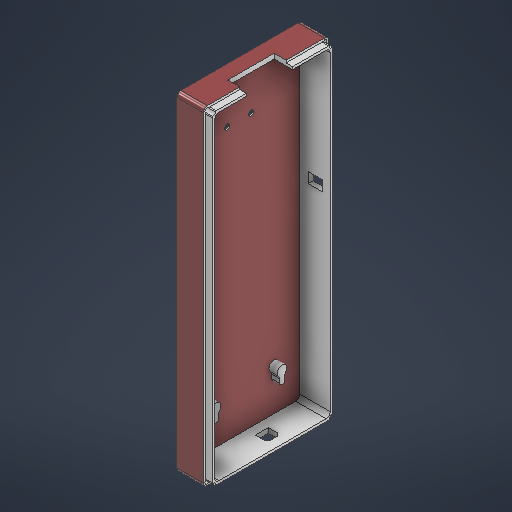
# Autodesk Inventor part: cDAQ_Bottom_Box3
Saved by Autodesk Inventor 2027 (Build 310192000, 192)
## iProperties
Created: 2026-05-08
Part Number: cDAQ_Bottom_Box3
Material: Generic
Document SubType Name: Modeling
Designer: giese
Density: 1 g/cm^3
Appearance: Default
Author: giese
Autodesk Inventor part; units mm, degrees
ref_plane "YZ Plane" through (0, 0, 0) normal (1, 0, 0) x (0, 1, 0)
ref_plane "XZ Plane" through (0, 0, 0) normal (0, 1, 0) x (-1, 0, 0)
ref_plane "XY Plane" through (0, 0, 0) normal (0, 0, 1) x (1, 0, 0)
sketch "Sketch1" plane through (0, 0, 0) normal (1, 0, 0) x (0, 1, 0)
  line L0 (37.5698, 48.0867) -> (-215.7952, 48.0867)
  line L1 (-215.7952, 48.0867) -> (-215.7952, -48.4333)
  line L2 (-215.7952, -48.4333) -> (37.5698, -48.4333)
  line L3 (37.5698, -48.4333) -> (37.5698, 48.0867)
  point P0 (0, 0)
  dimension "d0" = 96.52
  dimension "d1" = 253.365
  constraints: 8 end point, 2 parallel, 1 horizontal, 1 perpendicular
  measures "d0" distance of L2.end L0.start
  measures "d1" distance of L1.end L2.end
extrude "Extrusion1" add sketch "Sketch1" along normal blind 20.32
sketch "Sketch2" plane through (20.32, 0, 0) normal (1, 0, 0) x (0, 0, -1)
  line L0 (44.6233, 33.7598) -> (-44.2767, 33.7598)
  line L1 (-44.2767, 33.7598) -> (-44.2767, -211.9852)
  line L2 (-44.2767, -211.9852) -> (44.6233, -211.9852)
  line L3 (44.6233, -211.9852) -> (44.6233, 33.7598)
  line L4 (48.4333, 37.5698) -> (-48.0867, 37.5698) projected
  line L5 (-48.0867, 37.5698) -> (-48.0867, -215.7952) projected
  point P0 (0, 0)
  dimension "d4" = 245.745
  dimension "d5" = 88.9
  dimension "d8" = 3.81
  dimension "d21" = 3.81
  constraints: 8 end point, 2 parallel, 1 horizontal, 1 perpendicular
  measures "d4" distance of L2.end L0.start
  measures "d5" distance of L0.start L0.end
  measures "d8" distance between parallel lines of L0 L4
  measures "d21" distance between parallel lines of L5 L1
extrude "Extrusion2" cut sketch "Sketch2" against normal blind 18.415
sketch "Sketch3" plane through (0, 0, 0) normal (-1, 0, 0) x (0, 0, 1)
  circle A0 centre (-7.1989, -2.6638) radius 2
  circle A1 centre (11.2999, -2.6638) radius 2
  circle A2 centre (29.7987, -2.6638) radius 2
  line L0 (-48.4333, -215.7952) -> (-48.4333, 37.5698) projected
  line L1 (-48.4333, 37.5698) -> (48.0867, 37.5698) projected
  line L2 (48.0867, 37.5698) -> (48.0867, -215.7952) projected
  line L3 (44.2767, 33.7598) -> (-44.6233, 33.7598) projected
  point P0 (0, 0)
  point P1 (-0.896, -23.7433)
  point P2 (-45.1848, 27.0137)
  dimension "d9" = 18.4988
  dimension "d10" = 4
  dimension "d11" = 4
  dimension "d12" = 18.4988
  dimension "d13" = 36.9976
  dimension "d18" = 18.288
  dimension "d22" = 4
  dimension "d58" = 40.2336
  constraints: 3 centre point
  measures "d9" distance of A0.centre A1.centre
  measures "d10" diameter of A1
  measures "d11" diameter of A2
  measures "d12" distance of A1.centre A2.centre
  measures "d13" distance of A0.centre A2.centre
  measures "d18" distance from line of L2 A2.centre
  measures "d22" diameter of A0
  measures "d58" distance from line of L1 A2.centre
extrude "Extrusion3" cut sketch "Sketch3" against normal blind 3.81
sketch "Sketch5" plane through (0, -215.7952, -48.4333) normal (0, 0, -1) x (-1, 0, 0)
  line L0 (-19.2532, 150.6728) -> (-8.5598, 150.6728)
  line L1 (-8.5598, 150.6728) -> (-8.5598, 158.6728)
  line L2 (-8.5598, 158.6728) -> (-19.2532, 158.6728)
  line L3 (-19.2532, 158.6728) -> (-19.2532, 150.6728)
  line L4 (0, 253.365) -> (-20.32, 253.365) projected
  line L5 (0, 0) -> (0, 253.365) projected
  point P0 (0, 215.7952)
  point P1 (-13.9065, 158.6728)
  point P2 (-13.9065, 150.6728)
  dimension "d28" = 10.6934
  dimension "d30" = 8
  dimension "d31" = 8.5598
  dimension "d34" = 102.6922
  constraints: 8 end point, 2 midpoint, 2 parallel, 1 horizontal, 1 perpendicular
  measures "d28" distance between parallel lines of L1 L3
  measures "d30" distance of point (-13.907, 158.673) point (-13.907, 150.673)
  measures "d31" distance between parallel lines of L5 L1
  measures "d34" distance between parallel lines of L4 L0
extrude "Extrusion4" cut sketch "Sketch5" against normal blind 24.13
sketch "Sketch6" plane through (0, -215.7952, -48.4333) normal (0, -1, 0) x (1, 0, 0)
  line L0 (16, 45.1284) -> (9, 45.1284)
  line L1 (9, 45.1284) -> (9, 35.1284)
  line L2 (9, 35.1284) -> (16, 35.1284)
  line L3 (0, 96.52) -> (0, 0) projected
  line L4 (18.24, 43.1283) -> (18.24, 37.1284)
  line L5 (16, 45.1284) -> (18.24, 43.1283)
  line L6 (18.24, 37.1284) -> (16, 35.1284)
  line L7 (0, 0) -> (20.32, 0) projected
  point P0 (0, 48.4333)
  point P1 (12.5, 45.1284)
  point P2 (12.5, 35.1284)
  dimension "d35" = 10
  dimension "d39" = 6
  dimension "d48" = 45.1284
  dimension "d49" = 18.24
  constraints: 12 end point, 2 midpoint, 1 horizontal, 1 parallel, 1 perpendicular, 1 vertical
  measures "d35" distance of point (12.5, 45.128) point (12.5, 35.128)
  measures "d39" distance of L4.start L4.end
  measures "d48" distance between parallel lines of L7 L0
  measures "d49" distance between parallel lines of L3 L4
extrude "Extrusion5" cut sketch "Sketch6" against normal blind 3.81
sketch "Sketch7" plane through (0, 37.5698, 48.0867) normal (0, 1, 0) x (1, 0, 0)
  line L0 (26.1366, 63.754) -> (11.1252, 63.754)
  line L1 (11.1252, 63.754) -> (11.1252, 28.194)
  line L2 (11.1252, 28.194) -> (26.1366, 28.194)
  line L3 (26.1366, 28.194) -> (26.1366, 63.754)
  line L4 (0, 0) -> (20.32, 0) projected
  line L5 (0, 96.52) -> (0, 0) projected
  line L6 (20.32, 96.52) -> (20.32, 0) projected
  point P0 (0, 48.0867)
  dimension "d51" = 35.56
  dimension "d52" = 28.194
  dimension "d55" = 11.1252
  dimension "d56" = 15.0114
  dimension "d57" = 5.8166
  constraints: 8 end point, 2 parallel, 1 horizontal, 1 perpendicular
  measures "d51" distance of L2.end L0.start
  measures "d52" distance between parallel lines of L4 L2
  measures "d55" distance between parallel lines of L5 L1
  measures "d56" distance between parallel lines of L3 L1
  measures "d57" distance between parallel lines of L6 L3
extrude "Extrusion6" cut sketch "Sketch7" against normal blind 7.62
fillet "Fillet1" radius 3.175 4 edges at (10.16, 37.5698, -48.4333) (10.16, 37.5698, 48.0867) (10.16, -215.7952, -48.4333) (10.16, -215.7952, 48.0867)
sketch "Sketch8" plane through (0, 0, 0) normal (-1, 0, 0) x (0, 0, 1)
  line L0 (-8.9705, -6.1944) -> (-5.4399, -6.1944)
  line L1 (-8.9705, 0.8668) -> (-5.4399, 0.8668)
  line L2 (-8.9705, -6.1944) -> (-11.0089, -2.6638)
  line L3 (-8.9705, 0.8668) -> (-11.0089, -2.6638)
  line L4 (-5.4399, -6.1944) -> (-3.4016, -2.6638)
  line L5 (-5.4399, 0.8668) -> (-3.4016, -2.6638)
  circle A0 centre (-7.1989, -2.6638) radius 2 projected
  line L6 (9.5283, -6.1944) -> (13.0589, -6.1944)
  line L7 (9.5283, 0.8668) -> (13.0589, 0.8668)
  line L8 (9.5283, -6.1944) -> (7.4899, -2.6638)
  line L9 (9.5283, 0.8668) -> (7.4899, -2.6638)
  line L10 (13.0589, -6.1944) -> (15.0973, -2.6638)
  line L11 (13.0589, 0.8668) -> (15.0973, -2.6638)
  circle A1 centre (11.2999, -2.6638) radius 2 projected
  line L12 (28.0271, -6.1944) -> (25.9887, -2.6638)
  line L13 (28.0271, 0.8668) -> (25.9887, -2.6638)
  line L14 (28.0271, -6.1944) -> (31.5577, -6.1944)
  line L15 (28.0271, 0.8668) -> (31.5577, 0.8668)
  line L16 (31.5577, -6.1944) -> (33.5961, -2.6638)
  line L17 (31.5577, 0.8668) -> (33.5961, -2.6638)
  circle A2 centre (29.7987, -2.6638) radius 2 projected
  point P0 (-7.2052, -6.1944)
  point P1 (11.2936, -6.1944)
  point P2 (29.7924, -6.1944)
  point P3 (-11.0089, -2.6638)
  point P4 (-3.4016, -2.6638)
  point P5 (15.0973, -2.6638)
  point P6 (7.4899, -2.6638)
  point P7 (33.5961, -2.6638)
  point P8 (25.9887, -2.6638)
  dimension "d60" = 7.0612
  dimension "d61" = 120
  dimension "d62" = 120
  dimension "d63" = 120
  dimension "d64" = 120
  dimension "d65" = 3.5306
  dimension "d66" = 3.5306
  dimension "d67" = 3.5306
  dimension "d68" = 3.5306
  dimension "d69" = 3.5306
  dimension "d70" = 3.5306
  dimension "d71" = 0
  dimension "d72" = 7.6074
  dimension "d73" = 3.81
  dimension "d74" = 0
  dimension "d75" = 7.0612
  dimension "d76" = 120
  dimension "d77" = 120
  dimension "d78" = 120
  dimension "d79" = 120
  dimension "d80" = 3.5306
  dimension "d81" = 3.5306
  dimension "d82" = 3.5306
  dimension "d83" = 3.5306
  dimension "d84" = 3.5306
  dimension "d85" = 3.5306
  dimension "d86" = 0
  dimension "d87" = 7.6074
  dimension "d91" = 0
  dimension "d92" = 3.81
  dimension "d93" = 7.0612
  dimension "d94" = 120
  dimension "d95" = 120
  dimension "d96" = 120
  dimension "d97" = 120
  dimension "d98" = 3.5306
  dimension "d99" = 3.5306
  dimension "d100" = 3.5306
  dimension "d101" = 3.5306
  dimension "d102" = 3.5306
  dimension "d103" = 3.5306
  dimension "d104" = 0
  dimension "d105" = 7.6074
  dimension "d108" = 0
  dimension "d109" = 3.81
  constraints: 36 end point, 6 horizontal, 3 midpoint
  measures "d60" distance from line of point (-7.205, -6.194) L1
  measures "d61" angle of L0 L2
  measures "d62" angle of L1 L3
  measures "d63" angle of L4 L0
  measures "d64" angle of L5 L1
  measures "d65" distance of L0.start L0.end
  measures "d66" distance of L1.start L1.end
  measures "d67" vertical distance of L1.start L3.end
  measures "d68" vertical distance of L0.start L2.end
  measures "d69" vertical distance of L1.end L5.end
  measures "d70" vertical distance of L0.end L4.end
  measures "d71" horizontal distance of L0.start L1.start
  measures "d72" distance of L4.end L2.end
  measures "d73" distance of A0.centre L2.end
  measures "d74" vertical distance of A0.centre L4.end
  measures "d75" distance from line of point (11.294, -6.194) L7
  measures "d76" angle of L6 L8
  measures "d77" angle of L7 L9
  measures "d78" angle of L10 L6
  measures "d79" angle of L11 L7
  measures "d80" distance of L8.start L6.end
  measures "d81" distance of L9.start L7.end
  measures "d82" vertical distance of L9.start L9.end
  measures "d83" vertical distance of L8.start L8.end
  measures "d84" vertical distance of L7.end L11.end
  measures "d85" vertical distance of L6.end L10.end
  measures "d86" horizontal distance of L8.start L9.start
  measures "d87" distance of L10.end L8.end
  measures "d91" vertical distance of A1.centre L8.end
  measures "d92" distance of A1.centre L8.end
  measures "d93" distance from line of point (29.792, -6.194) L15
  measures "d94" angle of L14 L12
  measures "d95" angle of L15 L13
  measures "d96" angle of L16 L14
  measures "d97" angle of L17 L15
  measures "d98" distance of L12.start L16.start
  measures "d99" distance of L15.start L15.end
  measures "d100" vertical distance of L15.start L13.end
  measures "d101" vertical distance of L12.start L12.end
  measures "d102" vertical distance of L15.end L17.end
  measures "d103" vertical distance of L16.start L16.end
  measures "d104" horizontal distance of L12.start L15.start
  measures "d105" distance of L16.end L12.end
  measures "d108" vertical distance of A2.centre L12.end
  measures "d109" distance of A2.centre L12.end
extrude "Extrusion7" cut sketch "Sketch8" against normal blind 0.9525 contours L2 L3 L1 L5 L4 L0 | A0 | L8 L9 L7 L11 L10 L6 | A1 | L12 L13 L15 L17 L16 L14 | A2
sketch "Sketch9" plane through (1.905, 0, 0) normal (1, 0, 0) x (0, 0, -1)
  arc A0 (27.3489, -182.3284) -> (21.8927, -182.3284) centre (24.6208, -179.8542) ccw
  line L0 (45.2583, 37.5698) -> (15.6673, 37.5698) projected
  line L1 (44.6233, 33.7598) -> (44.6233, -211.9852) projected
  arc A1 (22.7158, -187.4742) -> (26.5258, -187.4742) centre (24.6208, -187.4742) ccw
  line L2 (26.5258, -187.4742) -> (26.5258, -184.4614)
  line L3 (22.7158, -187.4742) -> (22.7158, -184.4614)
  arc A2 (27.3489, -182.3284) -> (26.5258, -184.4614) centre (29.7008, -184.4614) ccw
  arc A3 (22.7158, -184.4614) -> (21.8927, -182.3284) centre (19.5408, -184.4614) ccw
  arc A4 (-23.4511, -182.3284) -> (-28.9073, -182.3285) centre (-26.1792, -179.8542) ccw
  arc A5 (-28.0842, -187.4606) -> (-24.2742, -187.4742) centre (-26.1792, -187.4742) ccw
  line L4 (-24.2742, -187.4742) -> (-24.2742, -184.4614)
  line L5 (-28.0842, -187.4606) -> (-28.0842, -184.4614)
  arc A6 (-23.4511, -182.3284) -> (-24.2742, -184.4614) centre (-21.0992, -184.4614) ccw
  arc A7 (-28.0842, -184.4614) -> (-28.9073, -182.3285) centre (-31.2592, -184.4614) ccw
  line L6 (-19.8927, 37.5698) -> (-44.9117, 37.5698) projected
  line L7 (-44.2767, -211.9852) -> (-44.2767, 33.7598) projected
  point P0 (0, 0)
  point P1 (26.5258, -183.0063)
  point P2 (22.7158, -183.0063)
  point P3 (-24.2742, -183.0063)
  point P4 (-28.0842, -183.0063)
  dimension "d112" = 217.424
  dimension "d114" = 7.366
  dimension "d116" = 3.81
  dimension "d117" = 225.044
  dimension "d118" = 3.175
  dimension "d119" = 7.366
  dimension "d120" = 3.81
  dimension "d121" = 3.175
  dimension "d122" = 217.424
  dimension "d123" = 225.044
  dimension "d125" = 0
  dimension "d128" = 50.8
  dimension "d129" = 20.0025
  dimension "d130" = 0
  constraints: 20 point on circle, 8 centre point, 8 end point, 8 tangent, 4 point on line, 2 equal radius, 2 parallel, 2 vertical
  measures "d112" distance from line of L0 A0.centre
  measures "d114" diameter of A0
  measures "d116" diameter of A1
  measures "d117" distance from line of L0 A1.centre
  measures "d118" radius of A2
  measures "d119" diameter of A4
  measures "d120" diameter of A5
  measures "d121" radius of A6
  measures "d122" distance from line of A4.centre L6
  measures "d123" distance from line of L6 A5.centre
  measures "d125" horizontal distance of A5.centre A4.centre
  measures "d128" distance of A5.centre A1.centre
  measures "d129" distance from line of L1 A0.centre
  measures "d130" horizontal distance of A0.centre A1.centre
extrude "Extrusion8" add sketch "Sketch9" along normal blind 6.4008
sketch "Sketch10" plane through (20.32, 0, 0) normal (1, 0, 0) x (0, 0, -1)
  line L0 (44.6233, -211.9852) -> (-44.2767, -211.9852) projected
  line L1 (-44.2767, -211.9852) -> (-44.2767, 33.7598) projected
  line L2 (-44.2767, -211.9852) -> (-44.2767, -209.6992)
  line L3 (-46.2767, -211.4452) -> (-46.2767, -213.9852)
  line L4 (-46.2767, -213.9852) -> (-41.9907, -213.9852)
  line L5 (-44.2767, -211.9852) -> (-41.9907, -211.9852)
  line L6 (44.6233, -211.9852) -> (42.3373, -211.9852)
  line L7 (42.3373, -213.9852) -> (46.6233, -213.9852)
  line L8 (46.6233, -213.9852) -> (46.6233, -209.6992)
  line L9 (44.6233, 33.7598) -> (44.6233, -211.9852) projected
  line L10 (-44.2767, -209.6992) -> (-44.2767, 33.7598)
  line L11 (-44.2767, 33.7598) -> (44.6233, 33.7598) projected
  line L12 (-41.9907, 35.7598) -> (-46.2767, 35.7598)
  line L13 (-46.2767, 35.7598) -> (-46.2767, 29.7278)
  line L14 (42.3373, 33.7598) -> (44.6233, 33.7598)
  line L15 (46.6233, 31.4738) -> (46.6233, 35.7598)
  line L16 (46.6233, 35.7598) -> (42.3373, 35.7598)
  line L17 (-41.9907, -213.9852) -> (42.3373, -213.9852)
  line L18 (42.3373, -211.9852) -> (-41.9907, -211.9852)
  line L19 (46.6233, -209.6992) -> (46.6233, 31.4738)
  line L20 (44.6233, 31.4738) -> (44.6233, -209.6992)
  line L21 (42.3373, 33.7598) -> (-41.9907, 33.7598)
  line L22 (-41.9907, 35.7598) -> (42.3373, 35.7598)
  line L23 (-44.2767, -209.6992) -> (-44.2767, -209.6992)
  line L24 (-46.2767, 29.7278) -> (-46.2767, -211.4452)
  point P0 (-41.9907, -213.8582)
  point P1 (-44.4037, -209.6992)
  point P2 (-46.2767, 32.7438)
  point P3 (44.6233, 31.4738)
  point P4 (42.3373, 35.7598)
  dimension "d139" = 2
  dimension "d142" = 2
  dimension "d143" = 2
  dimension "d146" = 2
  dimension "d147" = 2
  dimension "d150" = 2
  dimension "d151" = 2
  dimension "d159" = 2
  constraints: 42 end point, 7 point on line, 4 perpendicular, 3 horizontal, 3 parallel, 2 vertical, 1 collinear, 1 midpoint
  measures "d139" distance between parallel lines of L0 L4
  measures "d142" distance between parallel lines of L6 L7
  measures "d143" distance between parallel lines of L9 L8
  measures "d146" distance from line of point (-46.277, 32.744) L1
  measures "d147" distance between parallel lines of L11 L12
  measures "d150" distance between parallel lines of L11 L16
  measures "d151" distance between parallel lines of L9 L15
  measures "d159" distance from line of L1 L3.start
extrude "Extrusion9" add sketch "Sketch10" along normal blind 5
sketch "Sketch11" plane through (20.32, 35.7598, 19.8927) normal (0, 1, 0) x (1, 0, 0)
  line L0 (0, 35.56) -> (-9.1948, 35.56) projected
  line L1 (5, 66.516) -> (5, -26.384) projected
  line L2 (0, 35.56) -> (5, 35.56)
  line L3 (5, 35.56) -> (5, 0)
  line L4 (5, 0) -> (0, 0)
  line L5 (0, 0) -> (0, 35.56)
  point P0 (-20.32, 19.8927)
  point P1 (2.5, 0)
  point P2 (2.5, 35.56)
  point P3 (5, 35.56)
  dimension "d156" = 35.56
  constraints: 8 end point, 2 midpoint, 2 parallel, 1 horizontal, 1 perpendicular, 1 point on line
  measures "d156" distance of point (2.5, 0) point (2.5, 35.56)
extrude "Extrusion10" cut sketch "Sketch11" against normal blind 9.8425
fillet "Fillet2" radius 3.175 8 edges at (22.82, 35.7598, -46.6233) (22.82, 35.7598, 46.2767) (22.82, -213.9852, 46.2767) (22.82, -213.9852, -46.6233) (13.6125, 33.7598, -44.6233) (13.6125, 33.7598, 44.2767) (13.6125, -211.9852, 44.2767) (13.6125, -211.9852, -44.6233)
sketch "Sketch13" plane through (25.32, 0, 0) normal (1, 0, 0) x (0, 0, -1)
  arc A0 (46.6233, 32.5848) -> (43.4483, 35.7598) centre (43.4483, 32.5848) ccw projected
  arc A1 (-43.1017, 35.7598) -> (-46.2767, 32.5848) centre (-43.1017, 32.5848) ccw projected
  circle A2 centre (-45.3344, 34.8421) radius 1.5
  arc A3 (43.4483, -213.9852) -> (46.6233, -210.8102) centre (43.4483, -210.8102) ccw projected
  circle A4 centre (45.681, -213.0676) radius 1.5
  arc A5 (-46.2767, -210.8102) -> (-43.1017, -213.9852) centre (-43.1017, -210.8102) ccw projected
  circle A6 centre (-45.3344, -213.0676) radius 1.5
  circle A7 centre (45.681, 34.8421) radius 1.5
  line L0 (-19.8927, 37.5698) -> (-44.9117, 37.5698) projected
  line L1 (-48.0867, 34.3948) -> (-48.0867, -212.6202) projected
  point P0 (0, 0)
  point P1 (-45.3468, 34.8298)
  dimension "d166" = 3
  dimension "d167" = 3
  dimension "d168" = 3
  dimension "d169" = 3
  dimension "d170" = 2.7399
  dimension "d171" = 2.7523
  constraints: 5 point on circle, 4 centre point
  measures "d166" diameter of A6
  measures "d167" diameter of A4
  measures "d168" diameter of A2
  measures "d169" diameter of A7
  measures "d170" distance from line of L0 point (-45.347, 34.83)
  measures "d171" distance from line of L1 A2.centre
extrude "Extrusion11" cut sketch "Sketch13" against normal blind 25.4
body "Solid1"
